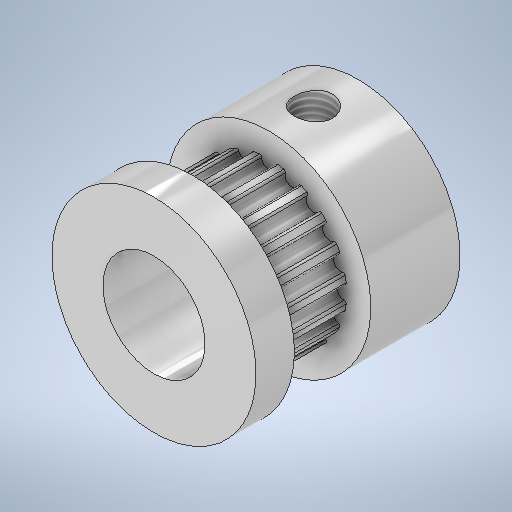
# Autodesk Inventor part: polea_GT2_8mm
Saved by Autodesk Inventor 2025.2 (Build 292293000, 293)
## iProperties
Created: 2023-10-01
Part Number: polea_GT2_8mm
Material: Genérico
Document SubType Name: Modeling
Designer: Samuel Pimentel
Density: 1 g/cm^3
Appearance: Aluminio - Pulido
Author: Samuel Pimentel
Autodesk Inventor part; units mm, degrees
ref_plane "YZ Plane" through (0, 0, 0) normal (1, 0, 0) x (0, 1, 0)
ref_plane "XY Plane" through (0, 0, 0) normal (0, 0, 1) x (1, 0, 0)
sketch "Boceto1" plane through (0, 0, 0) normal (0, 0, 1) x (1, 0, 0)
  line L0 (0, 4) -> (0, 8)
  line L1 (0, 8) -> (7, 8)
  line L2 (7, 8) -> (7, 5.362)
  line L3 (7, 5.362) -> (13, 5.362)
  line L4 (13, 5.362) -> (13, 8)
  line L5 (13, 8) -> (16, 8)
  line L6 (16, 8) -> (16, 4)
  line L7 (16, 0) -> (0, 0)
  line L8 (16, 4) -> (0, 4)
  dimension "d0" = 16
  dimension "d1" = 7
  dimension "d2" = 10.724
  dimension "d3" = 6
  dimension "d5" = 16
  dimension "d7" = 4
  constraints: 18 end point, 5 perpendicular, 2 horizontal, 2 point on line, 2 vertical alignment, 1 vertical
  measures "d0" diameter of L1 L7
  measures "d1" distance between parallel lines of L0 L2
  measures "d2" diameter of L3 L7
  measures "d3" distance between parallel lines of L4 L2
  measures "d5" distance between parallel lines of L0 L6
  measures "d7" distance between parallel lines of L8 L7
revolve "Revolución1" add sketch "Boceto1" angle 360 about axis through (16, 0, 0) along (-1, 0, 0)
sketch "Boceto2" plane through (7, 0, 0) normal (1, 0, 0) x (0, 0, -1)
  line L0 (0, 0) -> (0, 9) construction
  line L1 (0, 0) -> (1.4576, 9.2028) construction
  line L2 (0, 0) -> (2.9153, 8.9722) construction
  line L3 (0, 0) -> (2.1206, 9.4869) construction
  circle A0 centre (0, 0) radius 5.362 construction
  circle A1 centre (0, 0) radius 5.917 construction
  arc A2 (1.3014, 5.8013) -> (1.6569, 5.0996) centre (1.8285, 5.6274) ccw
  arc A3 (1.3014, 5.8013) -> (1.1881, 5.9954) centre (1.1589, 5.8483) ccw
  arc A4 (0, 5.362) -> (0.555, 5.9195) centre (0, 5.917) ccw
  arc A5 (0.7227, 6.0691) -> (0.555, 5.9195) centre (0.705, 5.9202) ccw
  arc A6 (1.1881, 5.9954) -> (0.7227, 6.0691) centre (0, 0) ccw
  arc A7 (-1.8887, -5.8129) -> (0, -6.112) centre (0, 0) ccw
  circle A8 centre (0, 0) radius 5.362
  point P0 (0, 5.362)
  dimension "d25" = 0.555
  dimension "d26" = 0.555
  dimension "d9" = 9
  dimension "d10" = 18
  dimension "d29" = 3.6
  dimension "d31" = 0.555
  dimension "d32" = 0.15
  dimension "d33" = 6.112
  constraints: 12 point on circle, 8 end point, 7 centre point, 5 symmetric about line, 3 point on line, 2 tangent, 1 coincident, 1 vertical, 8 other
  measures "d9" angle of L1 L0
  measures "d10" angle of L2 L0
  measures "d29" angle of L3 L1
  measures "d31" radius of A2
  measures "d32" radius of A3
  measures "d33" radius of A6
extrude "Extrusión1" add sketch "Boceto2" along normal up to surface (6 mm away) contours A2 A8 A4 A5 A6 A3
pattern_circular "Patrón circular1" count 20 over 360 about axis through (10, 0, 0) along (-1, 0, 0) of "Extrusión1"
ref_plane "Plano de trabajo1" through (3.5, 8, 0) normal (0, 1, 0) x (-1, 0, 0)
sketch "Boceto3" plane through (3.5, 8, 0) normal (0, 1, 0) x (-1, 0, 0)
  circle A0 centre (0, 0) radius 1.5
  line L0 (3.5, -8) -> (3.5, 8) projected
  line L1 (3.5, 0) -> (0, 0) construction
  dimension "d39" = 3
  dimension "d40" = 3.5
  constraints: 2 end point, 1 centre point, 1 horizontal
  measures "d39" diameter of A0
  measures "d40" distance from line of L1.end L0
extrude "Extrusión2" cut sketch "Boceto3" against normal up to surface
thread "Rosca1" size "M3x0.5" class "6H" standard "ANSI Metric M Profile" length 109.917
